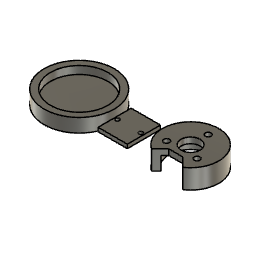
传感器安装底座 (Autodesk Fusion 360 design; units mm, degrees)
Autodesk Fusion 360 part; units mm, degrees
sketch "草图1" plane through (0, 0, 0) normal (0, 0, 1) x (1, 0, 0)
  circle A0 centre (-21.6844, 0.4639) radius 1.5
  circle A1 centre (-13.8344, 14.0605) radius 1.5
  circle A2 centre (-5.9844, 0.4639) radius 1.5
  dimension "d1" = 3
  dimension "d5" = 3
  dimension "d7" = 3
  measures "d1" diameter of A0
  measures "d5" diameter of A1
  measures "d7" diameter of A2
sketch "草图2" plane through (0, 0, 0) normal (0, 0, 1) x (1, 0, 0)
  circle A0 centre (-13.818, 4.9441) radius 14.5213
sketch "草图4" plane through (0, 0, 0) normal (0, 0, 1) x (1, 0, 0)
  circle A0 centre (-13.8325, 4.9588) radius 4.8825
extrude "拉伸1" add sketch "草图2" along normal blind 3 makes body 1
extrude "拉伸2" cut sketch "草图1" along normal blind 3 bodies 1
extrude "拉伸3" cut sketch "草图4" along normal blind 3 bodies 1
sketch "草图5" plane through (0, 0, 0) normal (0, 0, -1) x (1, 0, 0)
  circle A0 centre (-19.8325, -4.9588) radius 1
  circle A1 centre (-7.8325, -4.9588) radius 1
  line L0 (-21.4355, 3.5412) -> (-6.3219, 3.5412)
  line L1 (-6.3219, 3.5412) -> (-6.3219, -13.5319)
  line L2 (-6.3219, -13.5319) -> (-21.4355, -13.5319)
  line L3 (-21.4355, -13.5319) -> (-21.4355, 3.5412)
  dimension "d20" = 2
  dimension "d21" = 2
  constraint horizontal L0
  constraint vertical L1
  constraint horizontal L2
  constraint vertical L3
  measures "d20" diameter of A0
  measures "d21" diameter of A1
move_body "移动1" bodies 1 to x (1, 0, 0) y (0, 1, 0) z (0, 0, 1) at (-25.65, -0.2141, 0.0423)
extrude "拉伸4" add sketch "草图5" along normal blind 2 separate body makes body 2
sketch "草图6" plane through (0, 0, 0.0423) normal (0, 0, -1) x (1, 0, 0)
  circle A0 centre (-39.4825, -4.7447) radius 4.8825
  circle A1 centre (-39.4844, -13.8464) radius 1.5
  circle A2 centre (-31.6344, -0.2498) radius 1.5
  circle A3 centre (-47.3344, -0.2498) radius 1.5
  circle A4 centre (-39.468, -4.73) radius 14.5213
  circle A5 centre (-39.4825, -4.7447) radius 11.1034
  constraint concentric A0 A5
extrude "拉伸5" add sketch "草图6" along normal blind 7 contours A4 bodies 1
sketch "草图9" plane through (0, 0, 3.0423) normal (0, 0, 1) x (-1, 0, 0)
  circle A0 centre (39.4825, -4.7447) radius 4.8825
  circle A1 centre (39.4844, -13.8464) radius 1.5
  circle A2 centre (31.6344, -0.2498) radius 1.5
  circle A3 centre (47.3344, -0.2498) radius 1.5
  circle A4 centre (39.468, -4.73) radius 14.5213
  line L0 (43.3292, 2.7296) -> (47.7691, 7.1847)
  line L1 (43.3292, 2.7296) -> (36.1071, 2.7296)
  line L2 (36.1071, 2.7296) -> (31.4463, 7.3745)
  constraint coincident A4 L0.end
  constraint horizontal L1
  constraint coincident A4 L2.end
  constraint perpendicular L0 L2
extrude "拉伸6" cut sketch "草图9" against normal blind 11 contours A4 L0 L1 L2 picked at (39.691, 5.0832) bodies 1
sketch "草图10" plane through (0, 0, 0) normal (0, 0, 1) x (1, 0, 0)
  circle A0 centre (-39.4764, 4.7476) radius 18.074
  circle A1 centre (-39.4764, 4.7476) radius 14.7852
  constraint concentric A0 A1
move_body "移动2" bodies 1 to x (1, 0, 0) y (0, 1, 0) z (0, 0, 1) at (52.7735, 4.7608, 0)
extrude "拉伸7" add sketch "草图10" along normal blind 4 bodies 2
sketch "草图11" plane through (0, 0, 0) normal (0, 0, -1) x (1, 0, 0)
  line L0 (-21.4355, -5.8407) -> (-21.4355, -3.6545)
  arc A0 (-21.4355, -3.6545) -> (-21.4355, -5.8407) centre (-39.4764, -4.7476) ccw
  circle A1 centre (-39.4764, -4.7476) radius 14.7852
  circle A2 centre (-39.4764, -4.7476) radius 18.074
  constraint concentric A0 A2
extrude "拉伸8" add sketch "草图11" along normal blind 3 separate body contours A1 makes body 3
extrude "拉伸9" add 1 faces at (-22.6937, 7.0861, 0) along direction (0, 0, -1) blind 3 on bodies 2 bodies 2 3
